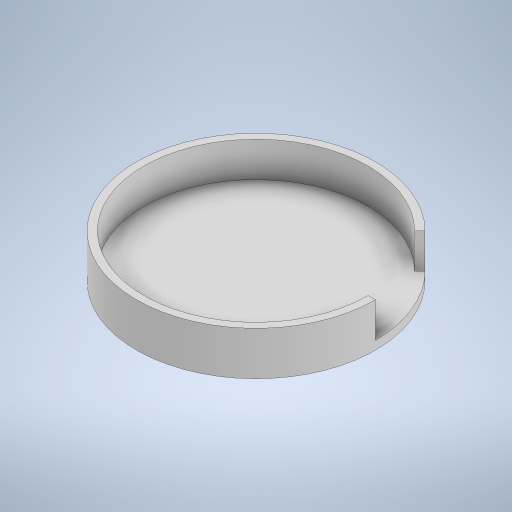
# Autodesk Inventor part: mainbody
Saved by Autodesk Inventor 2024 (Build 280153000, 153)
## iProperties
Created: 2024-05-20
Part Number: mainbody
Material: Generic
Document SubType Name: Modeling
Designer: ryana
Density: 1 g/cm^3
Appearance: Default
Author: ryana
Autodesk Inventor part; units mm, degrees
ref_plane "YZ Plane" through (0, 0, 0) normal (1, 0, 0) x (0, 1, 0)
ref_plane "XZ Plane" through (0, 0, 0) normal (0, 1, 0) x (-1, 0, 0)
ref_plane "XY Plane" through (0, 0, 0) normal (0, 0, 1) x (1, 0, 0)
sketch "Sketch1" plane through (0, 0, 0) normal (0, 1, 0) x (-1, 0, 0)
  circle A0 centre (0, 0) radius 38.5
  circle A1 centre (0, 0) radius 41
  dimension "d0" = 77
  dimension "d1" = 82
  constraints: 2 centre point, 2 coincident
  measures "d0" diameter of A0
  measures "d1" diameter of A1
extrude "Extrusion3" add sketch "Sketch1" along normal blind 3 contours A0
sketch "Sketch3" plane through (0, 0, 0) normal (0, 1, 0) x (-1, 0, 0)
  circle A0 centre (0, 0) radius 41
  circle A1 centre (0, 0) radius 38.5
  dimension "d9" = 82
  dimension "d10" = 77
  constraints: 2 centre point, 2 coincident
  measures "d9" diameter of A0
  measures "d10" diameter of A1
extrude "Extrusion4" add sketch "Sketch3" along normal blind 15
sketch "Sketch4" plane through (0, 3, 0) normal (0, 1, 0) x (1, 0, 0)
  line L0 (0, 0) -> (41, 0)
  circle A0 centre (0, 0) radius 41 projected
  line L1 (0, 0) -> (28.9914, 28.9914)
  line L2 (0, 0) -> (41, 0) construction
  arc A1 (41, 0) -> (28.9914, 28.9914) centre (0, 0) ccw
  dimension "d13" = 41
  dimension "d14" = 45
  constraints: 6 end point, 2 horizontal, 2 point on circle, 1 centre point, 1 equal length, 3 other
  measures "d13" distance of L0.start L1.end
  measures "d14" angle of L2 L1
extrude "Extrusion5" cut sketch "Sketch4" along normal blind 15 contours L1 A0 L0 picked at (21.0272, 17.2566)
body "Solid2"
